Autodesk Fusion 360 part; units mm, degrees
(part 2 of 2)
  spline S110 degree 3 poles (29.3716, 5.2937) (29.4328, 5.2987) (29.5558, 5.3088) (29.6585, 5.3774) (29.71, 5.4119) knots 0 0 0 0 0.018102 0.036374 0.036374 0.036374 0.036374
  spline S111 degree 3 poles (29.71, 5.4119) (29.7609, 5.46) (29.8723, 5.5653) (29.9342, 5.706) (29.9678, 5.7825) knots 0 0 0 0 0.020804 0.045551 0.045551 0.045551 0.045551
  spline S112 degree 3 poles (29.9678, 5.7825) (29.9978, 5.8777) (30.0869, 6.1604) (30.1638, 6.4466) (30.2149, 6.6365) knots 0 0 0 0 0.029943 0.088911 0.088911 0.088911 0.088911
  spline S113 degree 3 poles (30.2149, 6.6365) (30.2924, 6.9285) (30.4209, 7.4123) (30.5945, 7.8817) (30.6634, 8.0679) knots 0 0 0 0 0.090571 0.150073 0.150073 0.150073 0.150073
  spline S114 degree 3 poles (30.6634, 8.0679) (30.7268, 8.1948) (30.851, 8.4432) (31.0659, 8.6186) (31.1709, 8.7043) knots 0 0 0 0 0.042051 0.082236 0.082236 0.082236 0.082236
  spline S115 degree 3 poles (31.1709, 8.7043) (31.2926, 8.7716) (31.5496, 8.9138) (31.8434, 8.9279) (31.9981, 8.9353) knots 0 0 0 0 0.041152 0.086904 0.086904 0.086904 0.086904
  spline S116 degree 3 poles (31.9981, 8.9353) (32.1579, 8.9228) (32.4825, 8.8976) (32.7651, 8.7355) (32.9085, 8.6533) knots 0 0 0 0 0.047456 0.096374 0.096374 0.096374 0.096374
  spline S117 degree 3 poles (32.9085, 8.6533) (33.044, 8.5461) (33.3244, 8.3242) (33.4857, 8.0047) (33.5691, 7.8396) knots 0 0 0 0 0.051187 0.105937 0.105937 0.105937 0.105937
  spline S118 degree 3 poles (33.5691, 7.8396) (33.6372, 7.6526) (33.7788, 7.2642) (33.7946, 6.8509) (33.8028, 6.6365) knots 0 0 0 0 0.059313 0.123228 0.123228 0.123228 0.123228
  line L39 (31.4234, 28.6204) -> (33.6739, 27.1218)
  line L40 (33.6739, 27.1218) -> (33.6739, 25.9509)
  line L41 (33.6739, 25.9509) -> (30.709, 28.0349)
  line L42 (30.709, 28.0349) -> (27.9698, 26.1067)
  line L43 (27.9698, 26.1067) -> (27.9698, 27.3152)
  line L44 (27.9698, 27.3152) -> (29.3072, 28.1907)
  spline S119 degree 3 poles (29.3072, 28.1907) (29.4235, 28.2657) (29.6344, 28.4017) (29.8498, 28.5304) (29.9463, 28.5881) knots 0 0 0 0 0.041534 0.075271 0.075271 0.075271 0.075271
  spline S120 degree 3 poles (29.9463, 28.5881) (29.8345, 28.6632) (29.6229, 28.8052) (29.4156, 28.9533) (29.3179, 29.0232) knots 0 0 0 0 0.040409 0.076436 0.076436 0.076436 0.076436
  line L45 (29.3179, 29.0232) -> (27.9698, 29.9846)
  line L46 (27.9698, 29.9846) -> (27.9698, 31.1394)
  line L47 (27.9698, 31.1394) -> (30.6553, 29.1682)
  line L48 (30.6553, 29.1682) -> (33.6739, 31.2898)
  line L49 (33.6739, 31.2898) -> (33.6739, 30.1028)
  line L50 (33.6739, 30.1028) -> (31.9014, 28.9319)
  line L51 (31.9014, 28.9319) -> (31.4234, 28.6204)
  line L52 (25.7998, -8.5315) -> (33.6739, -8.5315)
  line L53 (33.6739, -8.5315) -> (33.6739, -9.4983)
  line L54 (33.6739, -9.4983) -> (25.7998, -9.4983)
  line L55 (25.7998, -9.4983) -> (25.7998, -8.5315)
  spline S121 degree 3 poles (33.8028, -19.0427) (33.7933, -19.3777) (33.7763, -19.9826) (33.4752, -20.5045) (33.3409, -20.7373) knots 0 0 0 0 0.098634 0.178087 0.178087 0.178087 0.178087
  spline S122 degree 3 poles (33.3409, -20.7373) (33.1603, -20.9153) (32.7764, -21.2936) (32.25, -21.4163) (31.9712, -21.4812) knots 0 0 0 0 0.074607 0.158576 0.158576 0.158576 0.158576
  line L56 (31.9712, -21.4812) -> (31.8208, -20.5252)
  spline S123 degree 3 poles (31.8208, -20.5252) (31.9981, -20.4899) (32.3348, -20.4229) (32.5838, -20.1879) (32.7017, -20.0767) knots 0 0 0 0 0.052996 0.100641 0.100641 0.100641 0.100641
  spline S124 degree 3 poles (32.7017, -20.0767) (32.7908, -19.9336) (32.9861, -19.6201) (33.0002, -19.2495) (33.0079, -19.0481) knots 0 0 0 0 0.049728 0.108971 0.108971 0.108971 0.108971
  spline S125 degree 3 poles (33.0079, -19.0481) (33.0033, -18.8494) (32.9951, -18.4955) (32.8154, -18.1926) (32.7366, -18.0598) knots 0 0 0 0 0.058403 0.104011 0.104011 0.104011 0.104011
  spline S126 degree 3 poles (32.7366, -18.0598) (32.645, -17.9659) (32.4689, -17.7854) (32.2197, -17.7531) (32.1001, -17.7376) knots 0 0 0 0 0.038117 0.073227 0.073227 0.073227 0.073227
  spline S127 degree 3 poles (32.1001, -17.7376) (31.9964, -17.75) (31.7863, -17.7751) (31.6523, -17.9392) (31.5845, -18.0222) knots 0 0 0 0 0.030125 0.060991 0.060991 0.060991 0.060991
  spline S128 degree 3 poles (31.5845, -18.0222) (31.5331, -18.1368) (31.3904, -18.4545) (31.309, -18.7936) (31.2569, -19.0105) knots 0 0 0 0 0.037608 0.104304 0.104304 0.104304 0.104304
  spline S129 degree 3 poles (31.2569, -19.0105) (31.1811, -19.3131) (31.0556, -19.8141) (30.867, -20.2946) (30.7923, -20.4849) knots 0 0 0 0 0.093451 0.15472 0.15472 0.15472 0.15472
  spline S130 degree 3 poles (30.7923, -20.4849) (30.7225, -20.6124) (30.5871, -20.86) (30.3599, -21.027) (30.2498, -21.1079) knots 0 0 0 0 0.043018 0.083508 0.083508 0.083508 0.083508
  spline S131 degree 3 poles (30.2498, -21.1079) (30.1307, -21.1698) (29.8907, -21.2946) (29.6206, -21.3115) (29.4844, -21.3201) knots 0 0 0 0 0.039778 0.080209 0.080209 0.080209 0.080209
  spline S132 degree 3 poles (29.4844, -21.3201) (29.3601, -21.3131) (29.1137, -21.2991) (28.8893, -21.1964) (28.7781, -21.1455) knots 0 0 0 0 0.036983 0.073328 0.073328 0.073328 0.073328
  spline S133 degree 3 poles (28.7781, -21.1455) (28.6744, -21.082) (28.4668, -20.955) (28.3145, -20.7652) (28.2383, -20.6702) knots 0 0 0 0 0.036186 0.072411 0.072411 0.072411 0.072411
  spline S134 degree 3 poles (28.2383, -20.6702) (28.1835, -20.583) (28.0625, -20.3907) (27.9939, -20.1738) (27.9563, -20.0552) knots 0 0 0 0 0.03077 0.0679 0.0679 0.0679 0.0679
  spline S135 degree 3 poles (27.9563, -20.0552) (27.9227, -19.9214) (27.8537, -19.6472) (27.8452, -19.3646) (27.8409, -19.22) knots 0 0 0 0 0.041269 0.084536 0.084536 0.084536 0.084536
  spline S136 degree 3 poles (27.8409, -19.22) (27.847, -19.0082) (27.8587, -18.6062) (27.9779, -18.2225) (28.0342, -18.041) knots 0 0 0 0 0.063228 0.119965 0.119965 0.119965 0.119965
  spline S137 degree 3 poles (28.0342, -18.041) (28.0997, -17.8865) (28.2215, -17.5991) (28.4515, -17.389) (28.5579, -17.2918) knots 0 0 0 0 0.049636 0.092371 0.092371 0.092371 0.092371
  spline S138 degree 3 poles (28.5579, -17.2918) (28.6838, -17.2165) (28.9578, -17.0526) (29.2717, -16.9917) (29.4414, -16.9588) knots 0 0 0 0 0.043668 0.095061 0.095061 0.095061 0.095061
  line L57 (29.4414, -16.9588) -> (29.5704, -17.9041)
  spline S139 degree 3 poles (29.5704, -17.9041) (29.4331, -17.9339) (29.1672, -17.9918) (28.9755, -18.1843) (28.8829, -18.2774) knots 0 0 0 0 0.04117 0.079724 0.079724 0.079724 0.079724
  spline S140 degree 3 poles (28.8829, -18.2774) (28.811, -18.3985) (28.652, -18.6664) (28.6415, -18.979) (28.6358, -19.1502) knots 0 0 0 0 0.041615 0.092013 0.092013 0.092013 0.092013
  spline S141 degree 3 poles (28.6358, -19.1502) (28.6373, -19.3447) (28.64, -19.6799) (28.7922, -19.9764) (28.856, -20.1008) knots 0 0 0 0 0.057333 0.098767 0.098767 0.098767 0.098767
  spline S142 degree 3 poles (28.856, -20.1008) (28.9294, -20.1838) (29.0682, -20.3407) (29.2744, -20.3711) (29.3716, -20.3855) knots 0 0 0 0 0.032048 0.06061 0.06061 0.06061 0.06061
  spline S143 degree 3 poles (29.3716, -20.3855) (29.4328, -20.3805) (29.5558, -20.3704) (29.6585, -20.3018) (29.71, -20.2673) knots 0 0 0 0 0.018102 0.036374 0.036374 0.036374 0.036374
  spline S144 degree 3 poles (29.71, -20.2673) (29.7609, -20.2192) (29.8723, -20.1139) (29.9342, -19.9732) (29.9678, -19.8967) knots 0 0 0 0 0.020804 0.045551 0.045551 0.045551 0.045551
  spline S145 degree 3 poles (29.9678, -19.8967) (29.9978, -19.8015) (30.0869, -19.5188) (30.1638, -19.2326) (30.2149, -19.0427) knots 0 0 0 0 0.029943 0.088911 0.088911 0.088911 0.088911
  spline S146 degree 3 poles (30.2149, -19.0427) (30.2924, -18.7507) (30.4209, -18.2669) (30.5945, -17.7975) (30.6634, -17.6113) knots 0 0 0 0 0.090571 0.150073 0.150073 0.150073 0.150073
  spline S147 degree 3 poles (30.6634, -17.6113) (30.7268, -17.4844) (30.851, -17.236) (31.0659, -17.0606) (31.1709, -16.9749) knots 0 0 0 0 0.042051 0.082236 0.082236 0.082236 0.082236
  spline S148 degree 3 poles (31.1709, -16.9749) (31.2926, -16.9076) (31.5496, -16.7654) (31.8434, -16.7513) (31.9981, -16.7439) knots 0 0 0 0 0.041152 0.086904 0.086904 0.086904 0.086904
  spline S149 degree 3 poles (31.9981, -16.7439) (32.1579, -16.7564) (32.4825, -16.7816) (32.7651, -16.9436) (32.9085, -17.0259) knots 0 0 0 0 0.047456 0.096374 0.096374 0.096374 0.096374
  spline S150 degree 3 poles (32.9085, -17.0259) (33.044, -17.1331) (33.3244, -17.355) (33.4857, -17.6745) (33.5691, -17.8396) knots 0 0 0 0 0.051187 0.105937 0.105937 0.105937 0.105937
  spline S151 degree 3 poles (33.5691, -17.8396) (33.6372, -18.0266) (33.7788, -18.415) (33.7946, -18.8283) (33.8028, -19.0427) knots 0 0 0 0 0.059313 0.123228 0.123228 0.123228 0.123228
  line L58 (-53.5, 33) -> (-50, 33)
  line L59 (-45.3, 33) -> (-50, 33)
  line L60 (-45.3, 33) -> (-45.3, 38.5)
  line L61 (-50, 38.5) -> (-45.3, 38.5)
  line L62 (-50.5, 38.5) -> (-50, 38.5)
  spline S152 degree 3 poles (-53.5, 35.5) (-53.5, 35.5019) (-53.5, 35.5038) (-53.5, 35.5174) (-53.4999, 35.5289) (-53.4995, 35.5586) (-53.4991, 35.5765) (-53.4966, 35.6547) (-53.493, 35.7111) (-53.4824, 35.8316) (-53.4745, 35.8946) (-53.4477, 36.071) (-53.4229, 36.1823) (-53.3339, 36.5155) (-53.2321, 36.7744) (-52.9327, 37.2793) (-52.6291, 37.712) (-51.8648, 38.1828) (-51.6278, 38.2938) (-51.102, 38.4515) (-50.8137, 38.5) (-50.5, 38.5) knots 2.276139 2.276139 2.276139 2.276139 2.27748 2.27748 2.285611 2.285611 2.298696 2.298696 2.34377 2.34377 2.403333 2.403333 2.532046 2.532046 2.871283 2.871283 3.20126 3.20126 3.325115 3.325115 3.446159 3.446159 3.446159 3.446159
  line L63 (-53.5, 35.5) -> (-53.5, 33)
  line L64 (-50, -33) -> (-53.5, -33)
  line L65 (-53.5, -33) -> (-53.5, -35.5)
  spline S153 degree 3 poles (-50.5, -38.5) (-50.8077, -38.5) (-51.1158, -38.4527) (-51.8831, -38.2075) (-52.2526, -37.9659) (-52.7828, -37.4746) (-52.9768, -37.2195) (-53.21, -36.799) (-53.2847, -36.6314) (-53.378, -36.3536) (-53.411, -36.2361) (-53.4523, -36.0382) (-53.4674, -35.9511) (-53.4878, -35.7808) (-53.4937, -35.7069) (-53.4981, -35.6095) (-53.4989, -35.5842) (-53.4997, -35.5453) (-53.4999, -35.5322) (-53.5, -35.5128) (-53.5, -35.5064) (-53.5, -35.5) knots 1.370803 1.370803 1.370803 1.370803 1.470636 1.470636 1.628431 1.628431 1.762685 1.762685 1.841928 1.841928 1.887602 1.887602 1.915126 1.915126 1.937693 1.937693 1.945444 1.945444 1.949383 1.949383 1.951297 1.951297 1.951297 1.951297
  line L66 (-45.3, -38.5) -> (-50.5, -38.5)
  line L67 (-45.3, -38.5) -> (-45.3, -33)
  line L68 (-50, -33) -> (-45.3, -33)
  line L69 (-8, -38.5) -> (-8, -4)
  line L70 (-8, -4) -> (9, -4)
  line L71 (9, -4) -> (9, 38.5)
  line L72 (-53.5, -33) -> (-53.5, 33)
  line L73 (-41.1, 27) -> (-41.1, 33)
  line L74 (-53.5, 27) -> (-41.1, 27)
  line L75 (-53.5, -27) -> (-41.1, -27)
  line L76 (-41.1, -27) -> (-41.1, -33)
  line L77 (-53.5, -33) -> (-53.5, -27)
  line L78 (-53.5, 33) -> (-53.5, 27)
  line L79 (-41.1, 30) -> (-53.5, 30) construction
  line L80 (-41.1, 32.5) -> (-53.5, 32.5)
  line L81 (-53.5, 32.5) -> (-53.5, 27.5)
  line L82 (-53.5, 27.5) -> (-41.1, 27.5)
  line L83 (-41.1, 27.5) -> (-41.1, 32.5)
  line L84 (0, 0) -> (-53.5, 0) construction
  line L85 (-41.1, -32.5) -> (-53.5, -32.5)
  line L86 (-53.5, -27.5) -> (-41.1, -27.5)
  dimension "d202" = 1
  dimension "d203" = 1
  dimension "d204" = 1
  dimension "d211" = 5
  constraint coincident L13 L69.start
  constraint perpendicular L13 L69
  constraint perpendicular L21 L70
  constraint coincident L15 L71.end
  constraint perpendicular L15 L71
  constraint coincident L64.end L65.start
  constraint coincident L58.start L63.end
  constraint midpoint L73 L79.start
  constraint midpoint L78 L79.end
  constraint horizontal L80
  constraint vertical L81
  constraint horizontal L82
  constraint vertical L83
  constraint midpoint L79.start L83
  constraint midpoint L79.end L81
  constraint coincident L84.start origin
  constraint midpoint L72 L84.end
  constraint symmetric L80.start L84 L85.start
  constraint symmetric L80.end L84 L85.end
  constraint symmetric L81.end L84 L86.start
  constraint symmetric L82.end L84 L86.end
  measures "d69" distance of S38.end
  measures "d202" distance of L21 L69
  measures "d203" distance of L20 L70
  measures "d204" distance of L19 L71
  measures "d211" distance of L80.start L82.end
extrude "Extrude mounts" add sketch "Bottom (2)" against normal blind 10.4 separate body contours L72 L73 L78 L80 L81 L82 L83 | L72 L76 L77 L85 L86 makes body 3 at (49.3667, -27.5, 41.5333) makes body 4 at (49.3667, 27.5, 41.5333) in component "Moving Lid"
extrude "Extrude thickness" add sketch "Bottom (2)" along normal blind 2.6 separate body contours L0 L1 L2 L3 L15 L60 L71 | L0 L58 L59 L60 L61 L62 S152 L63 | L1 L58 L59 L72 L73 L78 L80 | L2 L3 L9 L10 L69 L70 L71 L72 L73 L74 L75 L76 L83 | L72 L73 L78 L80 L81 L82 L83 | L72 L73 L74 L78 L82 | L9 L10 L11 L12 L13 L67 L69 | L72 L75 L76 L77 L86 | L12 L64 L65 S153 L66 L67 L68 | L11 L64 L68 L72 L76 L77 L85 | L72 L76 L77 L85 L86 makes body 5 in component "Moving Lid"
chamfer "Chamfer upper edge" distance 1.2 angle 55 5 edges at (20.75, -38.5, 47.6) (53.0938, -37.0074, 47.6) (53.5, 0, 47.6) (52.708, 37.531, 47.6) (29.25, 38.5, 47.6) measured on face at (38.3333, 1.3333, 47.6) measured on face at (38.3333, 1.3333, 47.6) measured on face at (38.3333, 1.3333, 47.6) measured on face at (38.3333, 1.3333, 47.6) measured on face at (38.3333, 1.3333, 47.6) on bodies 5 in component "Moving Lid"
chamfer "Chamfer gap edge" distance 2.6 angle 30 2 edges at (-9, -17.25, 45) (8, 21.25, 45) measured on face at (-9, -9, 45.8667) measured on face at (8, 14.3333, 46.7333) on bodies 5 in component "Moving Lid"
sketch "Mount holes" plane through (0, -32.5, 0) normal (0, -1, 0) x (1, 0, 0) in component "Moving Lid"
  line L0 (53.5, 45) -> (41.1, 45)
  line L1 (41.1, 45) -> (41.1, 34.6)
  line L2 (41.1, 34.6) -> (53.5, 34.6)
  line L3 (53.5, 34.6) -> (53.5, 45)
  circle A0 centre (47.3, 38.8) radius 1.5
  circle A1 centre (47.3, 38.8) radius 2.25
  arc A2 (47.3, 32.6) -> (53.5, 38.8) centre (47.3, 38.8) ccw construction
  line L4 (47.3, 38.8) -> (53.5, 38.8) construction
  line L5 (47.3, 38.8) -> (47.3, 34.6) construction
  line L6 (41.1, 45) -> (53.5, 45)
  line L7 (53.5, 45) -> (53.5, 39.6)
  line L8 (48.5, 34.6) -> (46.1, 34.6)
  line L9 (41.1, 39.6) -> (41.1, 45)
  arc A3 (41.1, 39.6) -> (46.1, 34.6) centre (46.1, 39.6) ccw
  arc A4 (48.5, 34.6) -> (53.5, 39.6) centre (48.5, 39.6) ccw
  dimension "d214" = 0.75
  dimension "d215" = 5
  constraint coincident L3 A2.end
  constraint coincident A0.centre A1.centre
  constraint perpendicular L3 L4
  constraint midpoint L2 L5.end
  constraint coincident A2.end L4.end
  constraint horizontal L6
  constraint vertical L7
  constraint horizontal L8
  constraint vertical L9
  constraint coincident L0.end L1.start
  constraint tangent L9 A3
  constraint tangent L8 A3
  constraint tangent L8 A4
  constraint tangent L7 A4
  constraint equal A3 A4
  measures "d215" radius of A3
extrude "Cut mount holes" cut sketch "Mount holes" against normal up to surface (65 mm away) contours L2 L3 A4 | L1 L2 A3 | A0 | A1 bodies 3 4 in component "Moving Lid"
component "Box Base" placed x (1, 0, 0) y (0, 1, 0) z (0, 0, 1) at (0, 0, 0)
component "Fixed Lid" placed x (1, 0, 0) y (0, 1, 0) z (0, 0, 1) at (0, 0, 0)
component "Moving Lid" placed x (1, 0, 0) y (0, 1, 0) z (0, 0, 1) at (0, 0, 0)
equation "BoxBaseInternalWidth = 70 mm"
equation "BoxBaseInternalLength = 100 mm"
equation "BoxBaseWallThickness = 3.5 mm"
equation "BoxBaseRoundedCornerRadius = 3 mm"
equation "d5 = BoxBaseInternalLength"
equation "d6 = BoxBaseInternalWidth"
equation "d7 = BoxBaseInternalWidth + BoxBaseWallThickness + BoxBaseWallThickness"
equation "d8 = BoxBaseInternalLength + BoxBaseWallThickness + BoxBaseWallThickness"
equation "d9 = BoxBaseRoundedCornerRadius"
equation "BoxBaseHeight = 45 mm"
equation "d11 = BoxBaseHeight"
equation "BoxBaseBottomThickness = 2.4 mm"
equation "d14 = BoxBaseBottomThickness"
equation "BoxBaseBottomEdgeChamfer = 2 mm"
equation "d17 = BoxBaseBottomEdgeChamfer"
equation "FixedLidWidth = 40 mm"
equation "d19 = FixedLidWidth"
equation "BoxBaseFixedLidMountWidth = 9 mm"
equation "d28 = BoxBaseFixedLidMountWidth - BoxBaseWallThickness"
equation "d31 = d28"
equation "d32 = d29"
equation "BoxBaseFixedLidScrewHoleDiameter = 3 mm"
equation "d37 = d36"
equation "d38 = BoxBaseFixedLidScrewHoleDiameter"
equation "d39 = BoxBaseFixedLidScrewHoleDiameter"
equation "BoxBaseFixedLidScrewHoleDepth = 15 mm"
equation "d41 = -BoxBaseFixedLidScrewHoleDepth"
equation "BoxBaseFixedLidScrewHoleChamfter = 1 mm"
equation "d44 = BoxBaseFixedLidScrewHoleChamfter"
equation "BoxBaseBoardWidth = 26.5 mm"
equation "BoxBaseBoardLength = 35 mm"
equation "BoxBaseBoardWallSupportHeight = 7 mm"
equation "BoxBaseBoardWallSupportThickness = 2 mm"
equation "BoxBaseBoardBottomSupportHeight = 2 mm"
equation "d50 = BoxBaseBoardLength"
equation "d51 = BoxBaseBoardWidth"
equation "d52 = BoxBaseBoardWallSupportThickness"
equation "d53 = BoxBaseBoardWallSupportThickness"
equation "d54 = BoxBaseBoardWallSupportHeight"
equation "d56 = BoxBaseBoardBottomSupportWidth"
equation "d57 = BoxBaseBoardBottomSupportHeight"
equation "BoxBaseBoardUsbHoleWidth = 7.5 mm"
equation "BoxBaseBoardUsbHoleHeight = 3.2 mm"
equation "BoxBaseBoardUsbCableWidth = 12.5 mm"
equation "BoxBaseBoardUsbCableHeight = 8.2 mm"
equation "d69 = BoxBaseBoardUsbHoleWidth"
equation "d70 = BoxBaseBoardUsbHoleHeight"
equation "d71 = BoxBaseBoardUsbCableWidth"
equation "d72 = BoxBaseBoardUsbCableHeight"
equation "d74 = -( BoxBaseWallThickness - 1 mm )"
equation "d76 = BoxBaseBottomEdgeChamfer"
equation "BoxBaseBoardBottomSupportWidth = 4 mm"
equation "BoxBaseShaftScrewHoleDiameter = 3 mm"
equation "BoxBaseShaftScrewHeadHoleDiameter = 6.4 mm"
equation "BoxBaseShaftScrewHeadHoleDepth = 3.5 mm"
equation "d99 = BoxBaseShaftScrewHoleDiameter"
equation "d100 = BoxBaseShaftScrewHeadHoleDiameter"
equation "d101 = BoxBaseShaftScrewHeadHoleDiameter + BoxBaseShaftScrewHoleWallThickness + BoxBaseShaftScrewHoleWallThickness"
equation "BoxBaseShaftScrewHoleWallThickness = 3 mm"
equation "d103 = d101 / 2"
equation "d104 = d103"
equation "d110 = -BoxBaseShaftScrewHeadHoleDepth"
equation "d112 = -BoxBaseShaftScrewHeadHoleDepth"
equation "OpenLidMountWidth = 5 mm"
equation "d115 = OpenLidMountWidth + 1 mm"
equation "d123 = d104 + 2 mm"
equation "d124 = d123"
equation "d128 = -d101"
equation "FixedLidScrewHoleDiameter = BoxBaseFixedLidScrewHoleDiameter + 0.8 mm"
equation "d132 = FixedLidScrewHoleDiameter"
equation "d133 = FixedLidScrewHoleDiameter"
equation "d134 = FixedLidScrewHoleDiameter"
equation "d135 = FixedLidScrewHoleDiameter"
equation "LidThickness = 2.6 mm"
equation "FixedLidSwitchHoleDiameter = 6.7 mm"
equation "d138 = FixedLidSwitchHoleDiameter"
equation "FixedLidSwitchHoleDistance = 11.5 mm"
equation "d140 = FixedLidSwitchHoleDistance"
equation "FixedLidExtensionLength = 17 mm"
equation "d143 = FixedLidExtensionLength"
equation "FixedLidArmHoleWidth = 10 mm"
equation "d145 = FixedLidArmHoleWidth / 2"
equation "d146 = LidThickness"
equation "LidUpperEdgeChamfer = 1.2 mm"
equation "d149 = LidUpperEdgeChamfer"
equation "FixedLidSensorHoleDiameter = 6.2 mm"
equation "d152 = FixedLidSensorHoleDiameter"
equation "FixedLidSensorLength = 16 mm"
equation "FixedLidSensorWidth = 21 mm"
equation "FixedLidSensorSupportWallThickness = 2 mm"
equation "d156 = FixedLidSensorLength"
equation "d157 = FixedLidSensorWidth"
equation "d158 = -FixedLidSensorSupportWallThickness"
equation "FixedLidSensorHoleDistanceFromEdge = 5 mm"
equation "d160 = FixedLidSensorHoleDistanceFromEdge"
equation "FixedLidSensorSupportWallHeight = 4 mm"
equation "d162 = FixedLidSensorSupportWallHeight"
equation "MotorMountWidth = 5.4 mm"
equation "MotorMountHeight = 13 mm"
equation "MotorMountDepth = 8.5 mm"
equation "MotorMountHoleDiameter = 2.2 mm"
equation "MotorMountDistance = 23.2 mm"
equation "FixedLidMotorMountDistanceFromCenter = 15 mm"
equation "d170 = FixedLidMotorMountDistanceFromCenter"
equation "d171 = MotorMountDepth"
equation "d172 = MotorMountWidth"
equation "d173 = d170"
equation "d174 = d171"
equation "d175 = d172"
equation "d176 = MotorMountDistance"
equation "d177 = MotorMountHeight"
equation "d179 = MotorMountHoleDiameter"
equation "d180 = d179"
equation "MotorMountHoleDistanceFromEdge = 6.3 mm"
equation "d182 = MotorMountHoleDistanceFromEdge"
equation "d183 = d182"
equation "FixedLidSensorMountWidth = 4.3 mm"
equation "FixedLidSensorMountHeight = 1.6 mm"
equation "FixedLidSensorMountScrewHoleDiameter = 2.5 mm"
equation "d192 = MotorMountWidth"
equation "d193 = MotorMountWidth"
equation "d194 = MotorMountWidth"
equation "d195 = MotorMountWidth"
equation "d196 = FixedLidSensorMountScrewHoleDiameter"
equation "d197 = FixedLidSensorMountScrewHoleDiameter"
equation "d198 = FixedLidSensorMountHeight"
equation "OpenLidGap = 1.0 mm"
equation "OpenLidGapBottomChamfer = LidThickness"
equation "d202 = OpenLidGap"
equation "d203 = OpenLidGap"
equation "d204 = OpenLidGap"
equation "d205 = LidThickness"
equation "d207 = LidUpperEdgeChamfer"
equation "d209 = OpenLidGapBottomChamfer"
equation "d211 = OpenLidMountWidth"
equation "d212 = -( d101 - 2 mm )"
named bodies: "Base", "Fixed Lid"
